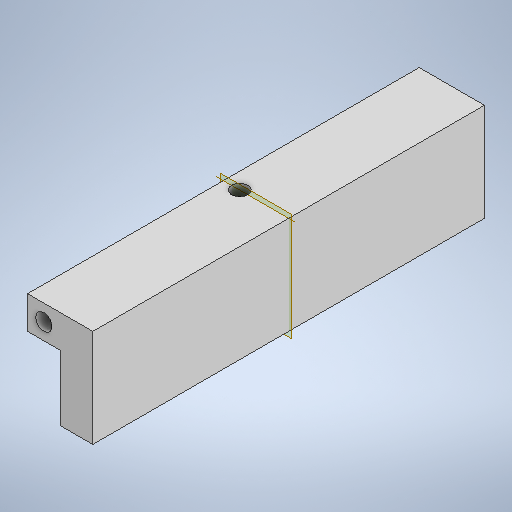
# Autodesk Inventor part: FuselageWingBoxJoint
Saved by Autodesk Inventor 2025.2 (Build 292293000, 293)
## iProperties
Created: 2025-04-12
Part Number: FuselageWingBoxJoint
Material: Generic
Document SubType Name: Modeling
Designer: georg
Density: 1 g/cm^3
Appearance: Default
Author: georg
Autodesk Inventor part; units mm, degrees
ref_plane "YZ Plane" through (0, 0, 0) normal (1, 0, 0) x (0, 1, 0)
ref_plane "XZ Plane" through (0, 0, 0) normal (0, 1, 0) x (-1, 0, 0)
ref_plane "XY Plane" through (0, 0, 0) normal (0, 0, 1) x (1, 0, 0)
sketch "Sketch1" plane through (0, 0, 0) normal (0, 0, 1) x (1, 0, 0)
  line L0 (0, 0) -> (10.7529, 0)
  line L1 (10.7529, 0) -> (10.7529, -25.4)
  line L2 (10.7529, -25.4) -> (23.4529, -25.4)
  line L3 (23.4529, -25.4) -> (23.4529, 12.7)
  line L4 (23.4529, 12.7) -> (-1.9471, 12.7)
  line L5 (-1.9471, 12.7) -> (-1.9471, 0)
  line L6 (-1.9471, 0) -> (10.7529, 0)
  dimension "d0" = 25.4
  dimension "d1" = 12.7
  dimension "d2" = 12.7
  dimension "d3" = 12.7
  constraints: 14 end point, 4 perpendicular, 2 horizontal, 1 vertical
  measures "d0" distance of L0.end L1.end
  measures "d1" distance of L1.end L2.end
  measures "d2" distance of L4.end L5.end
  measures "d3" distance of L5.end L0.end
extrude "Extrusion1" add sketch "Sketch1" along normal blind 152.4
sketch "Sketch2" plane through (-1.9471, 12.7, 0) normal (0, 1, 0) x (1, 0, 0)
  circle A0 centre (6.35, -76.2) radius 3.175
  line L0 (25.4, -152.4) -> (0, -152.4) projected
  line L1 (0, 0) -> (0, -152.4) projected
  point P0 (1.9471, 0)
  dimension "d6" = 6.35
  dimension "d7" = 76.2
  dimension "d8" = 6.35
  constraints: 1 centre point
  measures "d6" diameter of A0
  measures "d7" distance from line of L0 A0.centre
  measures "d8" distance from line of L1 A0.centre
extrude "Extrusion2" cut sketch "Sketch2" against normal blind 12.7
sketch "Sketch3" plane through (0, 0, 0) normal (0, 0, -1) x (-1, 0, 0)
  circle A0 centre (-4.4029, 6.35) radius 3.175
  line L0 (1.9471, 0) -> (-10.7529, 0) projected
  line L1 (1.9471, 12.7) -> (1.9471, 0) projected
  point P0 (0, 0)
  dimension "d11" = 6.35
  dimension "d12" = 6.35
  dimension "d13" = 6.35
  constraints: 1 centre point
  measures "d11" diameter of A0
  measures "d12" distance from line of L0 A0.centre
  measures "d13" distance from line of L1 A0.centre
extrude "Extrusion3" cut sketch "Sketch3" against normal blind 50.8
ref_plane "Work Plane1" through (-1.9471, 12.7, 76.2) normal (0, 0, -1) x (1, 0, 0)
mirror "Mirror1" about plane through (-1.9471, 12.7, 76.2) normal (0, 0, -1) of "Extrusion3"
body "Solid1"
